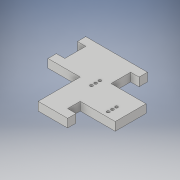
# Autodesk Inventor part: thumper-bumper-sidewall3-v3
Saved by Autodesk Inventor 2017 (Build 210142000, 142)
## iProperties
Created: 2017-02-22
Part Number: thumper-bumper-sidewall3-v3
Material: Generic
Document SubType Name: Modeling
Designer: John
Density: 1 g/cm^3
Appearance: Default
Author: John
Autodesk Inventor part; units mm, degrees
ref_plane "YZ Plane" through (0, 0, 0) normal (1, 0, 0) x (0, 1, 0)
ref_plane "XZ Plane" through (0, 0, 0) normal (0, 1, 0) x (-1, 0, 0)
ref_plane "XY Plane" through (0, 0, 0) normal (0, 0, 1) x (1, 0, 0)
sketch "Sketch1" plane through (0, 0, 0) normal (0, 1, 0) x (-1, 0, 0)
  line L0 (0, 0) -> (38, 0)
  line L1 (44, 0) -> (44, 6)
  line L2 (44, 27) -> (38, 27)
  line L3 (0, 27) -> (0, 6) construction
  line L4 (44, 27) -> (38, 27)
  line L5 (38, 27) -> (38, 21) construction
  line L6 (38, 21) -> (44, 21)
  line L7 (44, 21) -> (44, 27)
  line L8 (44, 0) -> (38, 0)
  line L9 (38, 0) -> (38, 6) construction
  line L10 (38, 6) -> (44, 6)
  line L11 (44, 6) -> (44, 0)
  line L12 (44, 21) -> (44, 27)
  line L13 (38, 27) -> (6, 27)
  line L14 (38, 0) -> (44, 0)
  line L15 (44, 6) -> (44, 21) construction
  line L16 (38, 6) -> (38, 21)
  line L17 (0, 0) -> (6, 0)
  line L18 (6, 0) -> (6, 6) construction
  line L19 (6, 6) -> (0, 6)
  line L20 (0, 6) -> (0, 0)
  line L21 (6, 6) -> (6, 27)
  line L22 (6, 27) -> (0, 27) construction
  line L23 (0, 6) -> (0, 0)
  line L24 (6, 27) -> (21, 27)
  line L25 (21, 27) -> (21, 57)
  line L26 (21, 57) -> (6, 57)
  line L27 (6, 57) -> (0, 57)
  line L28 (0, 57) -> (0, 51)
  line L29 (0, 51) -> (6, 51)
  line L30 (6, 51) -> (6, 57) construction
  line L31 (6, 51) -> (6, 27)
  line L32 (6, 42) -> (-19, 42)
  line L33 (-19, 42) -> (-19, 20)
  line L34 (-19, 20) -> (6, 20)
  line L35 (6, 20) -> (6, 42)
  dimension "d0" = 44
  dimension "d1" = 27
  dimension "d2" = 6
  dimension "d3" = 6
  dimension "d4" = 6
  dimension "d5" = 6
  dimension "d6" = 6
  dimension "d7" = 6
  dimension "d10" = 15
  dimension "d11" = 30
  dimension "d12" = 6
  dimension "d13" = 6
  dimension "d34" = 25
  dimension "d35" = 22
  dimension "d36" = 9
  constraints: 72 end point, 24 parallel, 14 perpendicular, 8 horizontal, 1 point on line
  measures "d0" distance of L3.start L2.start
  measures "d1" distance of L2.start L1.start
  measures "d2" distance of L6.end L5.end
  measures "d3" distance of L5.end L2.end
  measures "d4" distance of L9.end L1.end
  measures "d5" distance of L0.end L9.end
  measures "d6" distance of L3.end L18.end
  measures "d7" distance of L18.end L17.end
  measures "d10" distance of L26.end L25.end
  measures "d11" distance of L25.end L24.end
  measures "d12" distance of L29.end L28.end
  measures "d13" distance of L28.end L27.end
  measures "d34" distance of L34.end L33.end
  measures "d35" distance of L33.end L32.end
  measures "d36" distance between parallel lines of L32 L29
extrude "Extrusion1" add sketch "Sketch1" along normal blind 6
sketch "Sketch2" plane through (0, 6, 0) normal (0, 1, 0) x (1, 0, 0)
  circle A0 centre (10.5, -38.536) radius 1
  circle A1 centre (10.5, -35.536) radius 1
  circle A2 centre (10.5, -32.536) radius 1
  circle A3 centre (-11.7, -28.236) radius 1
  circle A4 centre (-11.7, -25.236) radius 1
  circle A5 centre (-11.7, -22.236) radius 1
  line L0 (0, -51) -> (-6, -51) projected
  line L1 (19, -42) -> (19, -20) projected
  dimension "d22" = 2
  dimension "d24" = 2
  dimension "d25" = 3
  dimension "d26" = 2
  dimension "d27" = 3
  dimension "d28" = 2
  dimension "d29" = 2
  dimension "d30" = 3
  dimension "d31" = 2
  dimension "d32" = 3
  dimension "d37" = 10.3
  dimension "d39" = 22.2
  dimension "d51" = 12.464
  dimension "d57" = 8.5
  constraints: 6 centre point
  measures "d22" diameter of A0
  measures "d24" diameter of A1
  measures "d25" distance of A1.centre A0.centre
  measures "d26" diameter of A2
  measures "d27" distance of A2.centre A1.centre
  measures "d28" diameter of A3
  measures "d29" diameter of A4
  measures "d30" distance of A4.centre A3.centre
  measures "d31" diameter of A5
  measures "d32" distance of A5.centre A4.centre
  measures "d37" vertical distance of A0.centre A3.centre
  measures "d39" horizontal distance of A0.centre A3.centre
  measures "d51" distance from line of A0.centre L0
  measures "d57" distance from line of L1 A0.centre
extrude "Extrusion2" cut sketch "Sketch2" against normal through all
body "Solid1"
